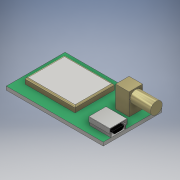
# Autodesk Inventor part: GPS
Saved by Autodesk Inventor 2016 (Build 200138000, 138)
## iProperties
Created: 2015-09-21
Part Number: GPS
Material: Generic
Document SubType Name: Modeling
Designer: lachesis
Density: 1 g/cm^3
Appearance: Default
Author: lachesis
Autodesk Inventor part; units mm, degrees
ref_plane "YZ Plane" through (0, 0, 0) normal (1, 0, 0) x (0, 1, 0)
ref_plane "XZ Plane" through (0, 0, 0) normal (0, 1, 0) x (-1, 0, 0)
ref_plane "XY Plane" through (0, 0, 0) normal (0, 0, 1) x (1, 0, 0)
sketch "Sketch1" plane through (0, 0, 0) normal (0, 1, 0) x (-1, 0, 0)
  line L0 (12.7, 20.955) -> (-12.7, 20.955)
  line L1 (-12.7, 20.955) -> (-12.7, -20.955)
  line L2 (-12.7, -20.955) -> (12.7, -20.955)
  line L3 (12.7, -20.955) -> (12.7, 20.955)
  point P0 (0, 0)
  point P1 (12.7, 0)
  point P2 (0, -20.955)
  dimension "d0" = 41.91
  dimension "d1" = 25.4
  constraints: 8 end point, 2 midpoint, 2 parallel, 1 horizontal, 1 horizontal alignment, 1 perpendicular, 1 vertical alignment
  measures "d0" distance of L2.end L0.start
  measures "d1" distance of L1.end L2.end
extrude "Extrusion1" add sketch "Sketch1" along normal blind 1.524
sketch "Sketch2" plane through (0, 1.524, 0) normal (0, 1, 0) x (1, 0, 0)
  line L0 (-9.144, -17.653) -> (7.874, -17.653)
  line L1 (7.874, -17.653) -> (7.874, 3.937)
  line L2 (7.874, 3.937) -> (-9.144, 3.937)
  line L3 (-9.144, 3.937) -> (-9.144, -17.653)
  line L4 (12.7, -20.955) -> (12.7, 20.955) projected
  line L5 (-12.7, -20.955) -> (12.7, -20.955) projected
  point P0 (0, 0)
  dimension "d4" = 21.59
  dimension "d5" = 17.018
  dimension "d6" = 4.826
  dimension "d7" = 3.302
  constraints: 8 end point, 2 parallel, 1 horizontal, 1 perpendicular
  measures "d4" distance of L2.end L0.start
  measures "d5" distance of L1.end L2.end
  measures "d6" distance between parallel lines of L4 L1
  measures "d7" distance between parallel lines of L0 L5
extrude "Extrusion2" add sketch "Sketch2" along normal blind 2.4384
fillet "Fillet1" radius 0.635 4 edges at (-0.635, 3.9624, 17.653) (7.874, 3.9624, 6.858) (-0.635, 3.9624, -3.937) (-9.144, 3.9624, 6.858)
sketch "Sketch3" plane through (0, 1.524, 0) normal (0, 1, 0) x (1, 0, 0)
  line L0 (-8.128, 11.303) -> (-2.286, 11.303)
  line L1 (-2.286, 11.303) -> (-2.286, 17.145)
  line L2 (-2.286, 17.145) -> (-8.128, 17.145)
  line L3 (-8.128, 17.145) -> (-8.128, 11.303)
  line L4 (-12.7, 20.955) -> (-12.7, -20.955) projected
  line L5 (12.7, 20.955) -> (-12.7, 20.955) projected
  point P0 (0, 0)
  dimension "d11" = 5.842
  dimension "d12" = 5.842
  dimension "d13" = 4.572
  dimension "d14" = 3.81
  constraints: 8 end point, 2 parallel, 1 horizontal, 1 perpendicular
  measures "d11" distance of L2.end L0.start
  measures "d12" distance of L0.start L0.end
  measures "d13" distance between parallel lines of L4 L3
  measures "d14" distance between parallel lines of L5 L2
extrude "Extrusion3" add sketch "Sketch3" along normal blind 9.398
sketch "Sketch4" plane through (-2.286, 1.524, -17.145) normal (0, 0, -1) x (-1, 0, 0)
  circle A0 centre (2.921, 6.35) radius 2.54
  line L0 (0, 9.398) -> (5.842, 9.398) projected
  point P0 (-2.286, -1.524)
  point P1 (2.921, 9.398)
  dimension "d17" = 5.08
  dimension "d18" = 0.508
  constraints: 1 centre point, 1 midpoint, 1 vertical alignment
  measures "d17" diameter of A0
  measures "d18" distance edge to line of A0 L0
extrude "Extrusion4" add sketch "Sketch4" along normal blind 8.89
sketch "Sketch5" plane through (12.7, 0, -20.955) normal (0, 0, -1) x (-1, 0, 0)
  line L0 (0, 1.524) -> (25.4, 1.524) projected
  line L1 (3.302, 1.524) -> (9.779, 1.524)
  line L2 (9.779, 1.524) -> (9.779, 3.048)
  line L3 (3.302, 3.048) -> (3.302, 1.524)
  line L4 (2.7305, 3.048) -> (2.7305, 5.1816)
  line L5 (2.7305, 5.1816) -> (10.3505, 5.1816)
  line L6 (10.3505, 5.1816) -> (10.3505, 3.048)
  line L7 (10.3505, 3.048) -> (9.779, 3.048)
  line L8 (3.302, 3.048) -> (2.7305, 3.048)
  point P0 (12.7, 0)
  point P1 (10.0648, 3.048)
  point P2 (3.0162, 3.048)
  dimension "d21" = 3.6576
  dimension "d22" = 1.524
  dimension "d23" = 7.62
  dimension "d24" = 6.477
  dimension "d25" = 3.302
  constraints: 16 end point, 4 parallel, 3 horizontal, 3 perpendicular, 2 midpoint, 1 collinear, 1 horizontal alignment, 1 point on line
  measures "d21" distance between parallel lines of L0 L5
  measures "d22" distance between parallel lines of L0 L8
  measures "d23" distance of L4.end L5.end
  measures "d24" distance between parallel lines of L2 L3
  measures "d25" distance from line of L0.start L3
extrude "Extrusion5" add sketch "Sketch5" against normal blind 9.017
sketch "Sketch6" plane through (12.7, 0, -20.955) normal (0, 0, -1) x (-1, 0, 0)
  line L0 (0, 0) -> (25.4, 0) projected
  line L1 (25.4, 0) -> (25.4, 1.524) projected
  line L2 (9.779, 1.524) -> (25.4, 1.524) projected
  line L3 (9.779, 1.524) -> (9.779, 3.048) projected
  line L4 (9.779, 3.048) -> (10.3505, 3.048) projected
  line L5 (10.3505, 3.048) -> (10.3505, 5.1816) projected
  line L6 (10.3505, 5.1816) -> (2.7305, 5.1816) projected
  line L7 (2.7305, 5.1816) -> (2.7305, 3.048) projected
  line L8 (2.7305, 3.048) -> (3.302, 3.048) projected
  line L9 (3.302, 3.048) -> (3.302, 1.524) projected
  line L10 (0, 1.524) -> (3.302, 1.524) projected
  line L11 (0, 0) -> (0, 1.524) projected
  line L12 (2.9845, 4.9276) -> (10.0965, 4.9276)
  line L13 (10.0965, 4.9276) -> (10.0965, 3.302)
  line L14 (2.9845, 3.302) -> (2.9845, 4.9276)
  line L15 (3.302, 1.524) -> (9.779, 1.524) projected
  line L16 (9.525, 3.302) -> (9.525, 1.524)
  line L17 (9.525, 1.524) -> (3.556, 1.524)
  line L18 (3.556, 1.524) -> (3.556, 3.302)
  line L19 (10.0965, 3.302) -> (9.525, 3.302)
  line L20 (3.556, 3.302) -> (2.9845, 3.302)
  line L21 (4.191, 3.5052) -> (8.89, 3.5052)
  line L22 (8.89, 3.5052) -> (8.89, 2.7686)
  line L23 (8.89, 2.7686) -> (4.191, 2.7686)
  line L24 (4.191, 2.7686) -> (4.191, 3.5052)
  line L25 (4.191, 2.7686) -> (4.9276, 2.032)
  line L26 (4.191, 2.7686) -> (5.2327, 2.7686) construction
  line L27 (4.9276, 2.032) -> (8.1534, 2.032)
  line L28 (8.1534, 2.032) -> (8.89, 2.7686)
  line L29 (6.5405, 3.5052) -> (6.5405, 2.032) construction
  point P0 (12.7, 0)
  point P1 (6.5405, 2.7686)
  point P2 (6.5405, 2.7686)
  dimension "d28" = 0.254
  dimension "d29" = 0.254
  dimension "d30" = 0.254
  dimension "d32" = 0.254
  dimension "d33" = 0.254
  dimension "d34" = 0.254
  dimension "d35" = 0.254
  dimension "d36" = 45
  dimension "d37" = 0.635
  dimension "d38" = 0.635
  dimension "d39" = 0.508
  dimension "d40" = 1.4224
  constraints: 34 end point, 7 parallel, 4 midpoint, 3 horizontal, 2 equal length, 2 perpendicular, 1 coincident, 1 point on line
  measures "d28" distance between parallel lines of L6 L12
  measures "d29" distance between parallel lines of L7 L14
  measures "d30" distance between parallel lines of L5 L13
  measures "d32" distance between parallel lines of L9 L18
  measures "d33" distance between parallel lines of L3 L16
  measures "d34" distance between parallel lines of L8 L20
  measures "d35" distance between parallel lines of L4 L19
  measures "d36" angle of L25 L26
  measures "d37" distance between parallel lines of L24 L18
  measures "d38" distance between parallel lines of L16 L22
  measures "d39" distance between parallel lines of L17 L27
  measures "d40" distance between parallel lines of L12 L21
extrude "Extrusion6" cut sketch "Sketch6" against normal blind 8.763 contours L18 L20 L14 L12 L13 L19 L16 L15
fillet "Fillet2" radius 0.127 10 edges at (9.9695, 3.048, -16.4465) (9.398, 3.048, -16.4465) (9.7155, 3.302, -16.5735) (9.144, 3.302, -16.5735) (3.175, 3.302, -16.5735) (2.6035, 3.302, -16.5735) (2.3495, 3.048, -16.4465) (2.921, 3.048, -16.4465) (2.3495, 5.1816, -16.4465) (9.9695, 5.1816, -16.4465)
equation "\"d12\" = d11"
equation "\"d29\" = d28"
equation "\"d30\" = d28"
equation "\"d32\" = d28"
equation "\"d33\" = d28"
equation "\"d34\" = d28"
equation "\"d35\" = d28"
equation "\"d38\" = d37"
equation "\"d31\" = d28"
body "Solid1"
